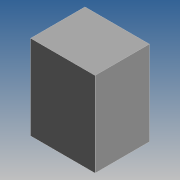
# Autodesk Inventor part: R004
Saved by Autodesk Inventor 2017 (Build 210142000, 142)
## iProperties
Created: 2018-10-05
Part Number: R004
Material: Générique
Document SubType Name: Modeling
Designer: Gilles Mottiez
Density: 1 g/cm^3
Appearance: Par défaut
Description: Port Ethernet Raspberry pi 3B
Author: Gilles Mottiez
Autodesk Inventor part; units mm, degrees
ref_plane "YZ Plane" through (0, 0, 0) normal (1, 0, 0) x (0, 1, 0)
ref_plane "XZ Plane" through (0, 0, 0) normal (0, 1, 0) x (-1, 0, 0)
ref_plane "XY Plane" through (0, 0, 0) normal (0, 0, 1) x (1, 0, 0)
sketch "Sketch1" plane through (0, 0, 0) normal (0, 0, 1) x (1, 0, 0)
  line L0 (0, 0) -> (16, 0)
  line L1 (16, 0) -> (16, 13.5)
  line L2 (16, 13.5) -> (0, 13.5)
  line L3 (0, 13.5) -> (0, 0)
  dimension "d0" = 16
  dimension "d1" = 13.5
  constraints: 8 end point, 2 parallel, 1 horizontal, 1 perpendicular
  measures "d0" distance of L2.end L1.end
  measures "d1" distance of L1.end L0.end
extrude "Extrusion1" add sketch "Sketch1" along normal blind 21
sketch "Esquisse3" plane through (0, 0, 0) normal (0, 0, -1) x (-1, 0, 0)
  line L0 (0, 0) -> (-16, 0) construction
  line L1 (0, 13.5) -> (0, 0) construction
  line L2 (-16, 13.5) -> (0, 13.5) construction
  line L3 (-16, 0) -> (-16, 13.5) construction
  line L4 (-14.5, 12.5) -> (-1.5, 12.5) construction
  line L5 (-1.5, 12.5) -> (-1.5, 4.5) construction
  line L6 (-1.5, 4.5) -> (-14.5, 4.5) construction
  line L7 (-14.5, 4.5) -> (-14.5, 12.5) construction
  line L8 (-5.5, 4.5) -> (-10.5, 4.5) construction
  line L9 (-10.5, 4.5) -> (-10.5, 1.5) construction
  line L10 (-10.5, 1.5) -> (-5.5, 1.5) construction
  line L11 (-5.5, 1.5) -> (-5.5, 4.5) construction
  line L12 (-8, 0) -> (-8, 13.5) construction
  line L13 (-14.5, 12.5) -> (-1.5, 12.5)
  line L14 (-1.5, 12.5) -> (-1.5, 4.5)
  line L15 (-1.5, 4.5) -> (-5.5, 4.5)
  line L16 (-5.5, 4.5) -> (-5.5, 1.5)
  line L17 (-5.5, 1.5) -> (-10.5, 1.5)
  line L18 (-10.5, 1.5) -> (-10.5, 4.5)
  line L19 (-10.5, 4.5) -> (-14.5, 4.5)
  line L20 (-14.5, 4.5) -> (-14.5, 12.5)
  dimension "d6" = 13
  dimension "d7" = 3
  dimension "d8" = 8
  dimension "d9" = 1
  dimension "d10" = 5
  constraints: 34 end point, 6 collinear, 5 parallel, 3 perpendicular, 2 horizontal, 2 midpoint, 1 point on line, 1 vertical, 2 other
  measures "d6" distance of L4.start L4.end
  measures "d7" distance of L10.end L8.start
  measures "d8" distance of L4.end L5.end
  measures "d9" distance between parallel lines of L2 L4
  measures "d10" distance of L9.end L10.end
extrude "Extrusion2" cut sketch "Esquisse3" against normal blind 19
